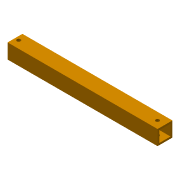
# Autodesk Inventor part: Yarm
Saved by Autodesk Inventor 2015 (Build 190159000, 159)
## iProperties
Created: 2015-01-13
Part Number: Yarm
Material: Generic
Document SubType Name: Modeling
Designer: Collin_2
Density: 1 g/cm^3
Appearance: Default
Author: Collin_2
Autodesk Inventor part; units mm, degrees
ref_plane "YZ Plane" through (0, 0, 0) normal (1, 0, 0) x (0, 1, 0)
ref_plane "XZ Plane" through (0, 0, 0) normal (0, 1, 0) x (-1, 0, 0)
ref_plane "XY Plane" through (0, 0, 0) normal (0, 0, 1) x (1, 0, 0)
sketch "Sketch1" plane through (0, 0, 0) normal (0, 1, 0) x (-1, 0, 0)
  line L0 (7.8808, 9.3738) -> (-248.8624, 9.3738)
  line L1 (-248.8624, 9.3738) -> (-248.8624, -16.0262)
  line L2 (-248.8624, -16.0262) -> (7.8808, -16.0262)
  line L3 (7.8808, -16.0262) -> (7.8808, 9.3738)
  point P0 (0, 0)
  dimension "d0" = 25.4
  dimension "d1" = 256.7432
  constraints: 8 end point, 2 parallel, 1 horizontal, 1 perpendicular
  measures "d0" distance of L2.end L0.start
  measures "d1" distance of L0.start L0.end
extrude "Extrusion1" add sketch "Sketch1" along normal blind 25.4
sketch "Sketch2" plane through (0, 25.4, 0) normal (0, 1, 0) x (1, 0, 0)
  line L0 (-7.8808, -9.3738) -> (248.8624, -9.3738)
  line L1 (248.8624, -9.3738) -> (248.8624, 16.0262)
  line L2 (248.8624, 16.0262) -> (-7.8808, 16.0262)
  line L3 (-7.8808, 16.0262) -> (-7.8808, -9.3738)
  circle A0 centre (-1.5308, 3.3262) radius 3.175
  circle A1 centre (236.1624, 3.3262) radius 3.175
  point P0 (0, 0)
  dimension "d4" = 6.35
  dimension "d5" = 6.35
  dimension "d6" = 237.6932
  dimension "d7" = 6.35
  constraints: 8 end point, 2 centre point, 2 parallel, 1 horizontal, 1 perpendicular
  measures "d4" diameter of A0
  measures "d5" diameter of A1
  measures "d6" distance of A1.centre A0.centre
  measures "d7" distance from line of L3 A0.centre
extrude "Extrusion2" cut sketch "Sketch2" against normal blind 25.4 contours A0 | A1
sketch "Sketch3" plane through (248.8624, 0, 9.3738) normal (1, 0, 0) x (0, 0, -1)
  line L0 (3.175, 22.225) -> (22.225, 22.225)
  line L1 (22.225, 22.225) -> (22.225, 3.175)
  line L2 (22.225, 3.175) -> (3.175, 3.175)
  line L3 (3.175, 3.175) -> (3.175, 22.225)
  line L4 (25.4, 0) -> (25.4, 25.4) projected
  line L5 (0, 25.4) -> (25.4, 25.4) projected
  line L6 (0, 0) -> (0, 25.4) projected
  line L7 (0, 0) -> (25.4, 0) projected
  point P0 (9.3738, 0)
  dimension "d10" = 3.175
  dimension "d11" = 3.175
  dimension "d12" = 3.175
  dimension "d13" = 3.175
  constraints: 8 end point, 2 parallel, 1 horizontal, 1 perpendicular
  measures "d10" distance between parallel lines of L4 L1
  measures "d11" distance between parallel lines of L5 L0
  measures "d12" distance between parallel lines of L6 L3
  measures "d13" distance between parallel lines of L7 L2
extrude "Extrusion3" cut sketch "Sketch3" against normal blind 228.6 contours L0 L1 L2 L3
body "Solid1"
